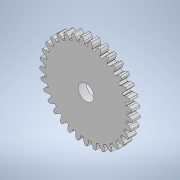
# Autodesk Inventor part: m1歯数33ギア3td6
Saved by Autodesk Inventor 2020.2 (Build 242310000, 310)
## iProperties
Created: 2020-02-29
Part Number: m1歯数33ギア3td6
Material: 一般
Document SubType Name: Modeling
Designer: aoyam
Density: 1 g/cm^3
Appearance: 既定
Author: aoyam
Autodesk Inventor part; units mm, degrees
ref_plane "YZ Plane" through (0, 0, 0) normal (1, 0, 0) x (0, 1, 0)
ref_plane "XZ Plane" through (0, 0, 0) normal (0, 1, 0) x (-1, 0, 0)
ref_plane "XY Plane" through (0, 0, 0) normal (0, 0, 1) x (1, 0, 0)
sketch "スケッチ1" plane through (0, 0, 0) normal (0, 0, 1) x (1, 0, 0)
  arc A0 (1.8965, 18.4525) -> (1.8679, 18.2509) centre (3.2757, 18.1542) ccw
  arc A1 (2.0839, 19.0802) -> (1.8965, 18.4525) centre (5.6844, 17.6636) ccw
  arc A2 (2.6531, 20.2065) -> (2.0839, 19.0802) centre (8.2766, 16.6576) ccw
  arc A3 (0.8542, 18.2509) -> (0.8257, 18.4525) centre (-0.5535, 18.1542) ccw
  arc A4 (0.8257, 18.4525) -> (0.6383, 19.0802) centre (-2.9622, 17.6636) ccw
  arc A5 (0.6383, 19.0802) -> (0.0691, 20.2065) centre (-5.5545, 16.6576) ccw
  arc A6 (1.8596, 17.9961) -> (0.8626, 17.9961) centre (1.3611, 2.7543) ccw
  arc A7 (0.0691, 20.2065) -> (-0.6732, 20.1356) centre (1.3611, 2.7543) ccw
  line L0 (1.8596, 17.9961) -> (1.8679, 18.2509)
  line L1 (0.8626, 17.9961) -> (0.8542, 18.2509)
  arc A8 (-1.0841, 18.2701) -> (-1.074, 18.0668) centre (0.3266, 18.2383) ccw
  arc A9 (-1.034, 17.815) -> (-2.013, 17.6263) centre (1.3611, 2.7543) ccw
  line L2 (-1.034, 17.815) -> (-1.074, 18.0668)
  line L3 (-2.013, 17.6263) -> (-2.0694, 17.8749)
  arc A10 (-2.0694, 17.8749) -> (-2.1356, 18.0675) centre (-3.4334, 17.5136) ccw
  arc A11 (-1.0189, 18.922) -> (-1.0841, 18.2701) centre (2.7846, 18.2124) ccw
  arc A12 (-2.1356, 18.0675) -> (-2.4384, 18.6484) centre (-5.7057, 16.576) ccw
  arc A13 (-0.6732, 20.1356) -> (-1.0189, 18.922) centre (5.5204, 17.7151) ccw
  arc A14 (-2.4384, 18.6484) -> (-3.2104, 19.6466) centre (-8.0607, 15.0976) ccw
  arc A15 (-3.2104, 19.6466) -> (-3.9258, 19.4365) centre (1.3611, 2.7543) ccw
  arc A16 (-3.9763, 17.527) -> (-3.9279, 17.3292) centre (-2.5851, 17.7627) ccw
  arc A17 (-3.8409, 17.0896) -> (-4.7666, 16.719) centre (1.3611, 2.7543) ccw
  line L4 (-3.8409, 17.0896) -> (-3.9279, 17.3292)
  line L5 (-4.7666, 16.719) -> (-4.869, 16.9525)
  arc A18 (-4.869, 16.9525) -> (-4.9704, 17.129) centre (-6.14, 16.3395) ccw
  arc A19 (-4.0356, 18.1794) -> (-3.9763, 17.527) centre (-0.1666, 18.2024) ccw
  arc A20 (-4.9704, 17.129) -> (-5.3777, 17.6421) centre (-8.1938, 14.9888) ccw
  arc A21 (-3.9258, 19.4365) -> (-4.0356, 18.1794) centre (2.6139, 18.2319) ccw
  arc A22 (-5.3777, 17.6421) -> (-6.3247, 18.4762) centre (-10.2265, 13.0914) ccw
  arc A23 (-6.3247, 18.4762) -> (-6.9874, 18.1345) centre (1.3611, 2.7543) ccw
  arc A24 (-6.6756, 16.2499) -> (-6.5907, 16.0649) centre (-5.3541, 16.7446) ccw
  arc A25 (-6.4599, 15.846) -> (-7.2987, 15.307) centre (1.3611, 2.7543) ccw
  line L6 (-6.4599, 15.846) -> (-6.5907, 16.0649)
  line L7 (-7.2987, 15.307) -> (-7.4434, 15.5168)
  arc A26 (-7.4434, 15.5168) -> (-7.5765, 15.671) centre (-8.5754, 14.6744) ccw
  arc A27 (-6.8573, 16.8793) -> (-6.6756, 16.2499) centre (-3.0625, 17.6342) ccw
  arc A28 (-7.5765, 15.671) -> (-8.0734, 16.0977) centre (-10.3365, 12.9595) ccw
  arc A29 (-6.9874, 18.1345) -> (-6.8573, 16.8793) centre (-0.3379, 18.1893) ccw
  arc A30 (-8.0734, 16.0977) -> (-9.1612, 16.7375) centre (-11.9734, 10.7117) ccw
  arc A31 (-9.1612, 16.7375) -> (-9.7473, 16.2766) centre (1.3611, 2.7543) ccw
  arc A32 (-9.0844, 14.4851) -> (-8.966, 14.3195) centre (-7.8805, 15.221) ccw
  arc A33 (-8.7962, 14.1293) -> (-9.5178, 13.4413) centre (1.3611, 2.7543) ccw
  line L8 (-8.7962, 14.1293) -> (-8.966, 14.3195)
  line L9 (-9.5178, 13.4413) -> (-9.6997, 13.6199)
  arc A34 (-9.6997, 13.6199) -> (-9.8594, 13.7461) centre (-10.6518, 12.5785) ccw
  arc A35 (-9.382, 15.0687) -> (-9.0844, 14.4851) centre (-5.7986, 16.5281) ccw
  arc A36 (-9.8594, 13.7461) -> (-10.4282, 14.0711) centre (-12.0565, 10.5613) ccw
  arc A37 (-9.7473, 16.2766) -> (-9.382, 15.0687) centre (-3.2283, 17.5889) ccw
  arc A38 (-10.4282, 14.0711) -> (-11.6174, 14.4935) centre (-13.2384, 8.0443) ccw
  arc A39 (-11.6174, 14.4935) -> (-12.1057, 13.93) centre (1.3611, 2.7543) ccw
  arc A40 (-11.1158, 12.2963) -> (-10.9681, 12.1561) centre (-10.0728, 13.2467) ccw
  arc A41 (-10.7654, 12.0015) -> (-11.3437, 11.1893) centre (1.3611, 2.7543) ccw
  line L10 (-10.7654, 12.0015) -> (-10.9681, 12.1561)
  line L11 (-11.3437, 11.1893) -> (-11.5561, 11.3303)
  arc A42 (-11.5561, 11.3303) -> (-11.7369, 11.424) centre (-12.2939, 10.1275) ccw
  arc A43 (-11.5184, 12.813) -> (-11.1158, 12.2963) centre (-8.276, 14.9242) ccw
  arc A44 (-11.7369, 11.424) -> (-12.3569, 11.6355) centre (-13.2915, 7.8809) ccw
  arc A45 (-12.1057, 13.93) -> (-11.5184, 12.813) centre (-5.9528, 16.4522) ccw
  arc A46 (-12.3569, 11.6355) -> (-13.6045, 11.8251) centre (-13.9757, 5.1858) ccw
  arc A47 (-13.6045, 11.8251) -> (-13.9773, 11.1794) centre (1.3611, 2.7543) ccw
  arc A48 (-12.6961, 9.7626) -> (-12.5246, 9.6528) centre (-11.8519, 10.8932) ccw
  arc A49 (-12.2963, 9.5394) -> (-12.7105, 8.6325) centre (1.3611, 2.7543) ccw
  line L12 (-12.2963, 9.5394) -> (-12.5246, 9.6528)
  line L13 (-12.7105, 8.6325) -> (-12.9457, 8.7308)
  arc A50 (-12.9457, 8.7308) -> (-13.141, 8.7885) centre (-13.4426, 7.4101) ccw
  arc A51 (-13.1893, 10.1938) -> (-12.6961, 9.7626) centre (-10.405, 12.8805) ccw
  arc A52 (-13.141, 8.7885) -> (-13.7898, 8.8788) centre (-13.9969, 5.0152) ccw
  arc A53 (-13.9773, 11.1794) -> (-13.1893, 10.1938) centre (-8.413, 14.8205) ccw
  arc A54 (-13.7898, 8.8788) -> (-15.0508, 8.829) centre (-14.1587, 2.2393) ccw
  arc A55 (-15.0508, 8.829) -> (-15.2946, 8.1243) centre (1.3611, 2.7543) ccw
  arc A56 (-13.7684, 6.9756) -> (-13.5792, 6.9003) centre (-13.1534, 8.2456) ccw
  arc A57 (-13.3336, 6.8321) -> (-13.5687, 5.8632) centre (1.3611, 2.7543) ccw
  line L14 (-13.3336, 6.8321) -> (-13.5792, 6.9003)
  line L15 (-13.5687, 5.8632) -> (-13.8182, 5.9152)
  arc A58 (-13.8182, 5.9152) -> (-14.0209, 5.9349) centre (-14.0562, 4.5243) ccw
  arc A59 (-14.3343, 7.3057) -> (-13.7684, 6.9756) centre (-12.1088, 10.4707) ccw
  arc A60 (-14.0209, 5.9349) -> (-14.6751, 5.9008) centre (-14.1473, 2.0678) ccw
  arc A61 (-15.2946, 8.1243) -> (-14.3343, 7.3057) centre (-10.52, 12.7527) ccw
  arc A62 (-14.6751, 5.9008) -> (-15.9038, 5.6132) centre (-13.7808, -0.6885) ccw
  arc A63 (-15.9038, 5.6132) -> (-16.0099, 4.8752) centre (1.3611, 2.7543) ccw
  arc A64 (-14.2939, 4.036) -> (-14.0939, 3.9979) centre (-13.9303, 5.3994) ccw
  arc A65 (-13.8398, 3.9775) -> (-13.8872, 2.9815) centre (1.3611, 2.7543) ccw
  line L16 (-13.8398, 3.9775) -> (-14.0939, 3.9979)
  line L17 (-13.8872, 2.9815) -> (-14.1421, 2.9853)
  arc A66 (-14.1421, 2.9853) -> (-14.3449, 2.9664) centre (-14.1125, 1.5746) ccw
  arc A67 (-14.912, 4.2531) -> (-14.2939, 4.036) centre (-13.3257, 7.7821) ccw
  arc A68 (-14.3449, 2.9664) -> (-14.9808, 2.8091) centre (-13.7371, -0.8547) ccw
  arc A69 (-16.0099, 4.8752) -> (-14.912, 4.2531) centre (-12.1975, 10.3235) ccw
  arc A70 (-14.9808, 2.8091) -> (-16.1329, 2.2942) centre (-12.8556, -3.4919) ccw
  arc A71 (-16.1329, 2.2942) -> (-16.0974, 1.5494) centre (1.3611, 2.7543) ccw
  arc A72 (-14.2536, 1.0501) -> (-14.05, 1.0506) centre (-14.1546, 2.4577) ccw
  arc A73 (-13.7966, 1.0786) -> (-13.6547, 0.0917) centre (1.3611, 2.7543) ccw
  line L18 (-13.7966, 1.0786) -> (-14.05, 1.0506)
  line L19 (-13.6547, 0.0917) -> (-13.9057, 0.0472)
  arc A74 (-13.9057, 0.0472) -> (-14.1012, -0.0098) centre (-13.6097, -1.3325) ccw
  arc A75 (-14.9016, 1.1463) -> (-14.2536, 1.0501) centre (-14.0118, 4.9117) ccw
  arc A76 (-14.1012, -0.0098) -> (-14.6958, -0.2846) centre (-12.7813, -3.6469) ccw
  arc A77 (-16.0974, 1.5494) -> (-14.9016, 1.1463) centre (-13.3849, 7.6208) ccw
  arc A78 (-14.6958, -0.2846) -> (-15.7297, -1.0083) centre (-11.4166, -6.0696) ccw
  arc A79 (-15.7297, -1.0083) -> (-15.5539, -1.7329) centre (1.3611, 2.7543) ccw
  arc A80 (-13.6489, -1.8742) -> (-13.449, -1.8352) centre (-13.8181, -0.4733) ccw
  arc A81 (-13.2055, -1.7598) -> (-12.8794, -2.702) centre (1.3611, 2.7543) ccw
  line L20 (-13.2055, -1.7598) -> (-13.449, -1.8352)
  line L21 (-12.8794, -2.702) -> (-13.1175, -2.7932)
  arc A82 (-13.1175, -2.7932) -> (-13.2986, -2.8861) centre (-12.5657, -4.0919) ccw
  arc A83 (-14.3034, -1.9024) -> (-13.6489, -1.8742) centre (-14.1423, 1.9634) ccw
  arc A84 (-13.2986, -2.8861) -> (-13.8306, -3.2685) centre (-11.3143, -6.2076) ccw
  arc A85 (-15.5539, -1.7329) -> (-14.3034, -1.9024) centre (-14.0395, 4.7421) ccw
  arc A86 (-13.8306, -3.2685) -> (-14.7087, -4.1747) centre (-9.5157, -8.3283) ccw
  arc A87 (-14.7087, -4.1747) -> (-14.399, -4.853) centre (1.3611, 2.7543) ccw
  arc A88 (-12.5017, -4.6312) -> (-12.3128, -4.5551) centre (-12.933, -3.2876) ccw
  arc A89 (-12.088, -4.4349) -> (-11.5895, -5.2984) centre (1.3611, 2.7543) ccw
  line L22 (-12.088, -4.4349) -> (-12.3128, -4.5551)
  line L23 (-11.5895, -5.2984) -> (-11.806, -5.433)
  arc A90 (-11.806, -5.433) -> (-11.9663, -5.5585) centre (-11.0184, -6.6038) ccw
  arc A91 (-13.139, -4.7828) -> (-12.5017, -4.6312) centre (-13.7125, -0.9563) ccw
  arc A92 (-11.9663, -5.5585) -> (-12.4162, -6.0347) centre (-9.3892, -8.4445) ccw
  arc A93 (-14.399, -4.853) -> (-13.139, -4.7828) centre (-14.1374, 1.7916) ccw
  arc A94 (-12.4162, -6.0347) -> (-13.107, -7.0907) centre (-7.2218, -10.1865) ccw
  arc A95 (-13.107, -7.0907) -> (-12.6745, -7.6981) centre (1.3611, 2.7543) ccw
  arc A96 (-10.8535, -7.1212) -> (-10.6824, -7.0108) centre (-11.5312, -5.8836) ccw
  arc A97 (-10.4844, -6.8503) -> (-9.8315, -7.6038) centre (1.3611, 2.7543) ccw
  line L24 (-10.4844, -6.8503) -> (-10.6824, -7.0108)
  line L25 (-9.8315, -7.6038) -> (-10.0186, -7.7769)
  arc A98 (-10.0186, -7.7769) -> (-10.1522, -7.9305) centre (-9.0236, -8.7775) ccw
  arc A99 (-11.4506, -7.3907) -> (-10.8535, -7.1212) centre (-12.7378, -3.742) ccw
  arc A100 (-10.1522, -7.9305) -> (-10.5039, -8.4832) centre (-7.0755, -10.2766) ccw
  arc A101 (-12.6745, -7.6981) -> (-11.4506, -7.3907) centre (-13.6751, -1.1241) ccw
  arc A102 (-10.5039, -8.4832) -> (-10.9824, -9.6509) centre (-4.6177, -11.5769) ccw
  arc A103 (-10.9824, -9.6509) -> (-10.4428, -10.1655) centre (1.3611, 2.7543) ccw
  arc A104 (-8.7638, -9.2544) -> (-8.6167, -9.1136) centre (-9.6635, -8.1674) ccw
  arc A105 (-8.4527, -8.9185) -> (-7.669, -9.5348) centre (1.3611, 2.7543) ccw
  line L26 (-8.4527, -8.9185) -> (-8.6167, -9.1136)
  line L27 (-7.669, -9.5348) -> (-7.8199, -9.7402)
  arc A106 (-7.8199, -9.7402) -> (-7.9221, -9.9164) centre (-6.6536, -10.5344) ccw
  arc A107 (-9.2991, -9.632) -> (-8.7638, -9.2544) centre (-11.2536, -6.2928) ccw
  arc A108 (-7.9221, -9.9164) -> (-8.1628, -10.5256) centre (-4.4569, -11.6378) ccw
  arc A109 (-10.4428, -10.1655) -> (-9.2991, -9.632) centre (-12.6694, -3.8996) ccw
  arc A110 (-8.1628, -10.5256) -> (-8.4116, -11.7628) centre (-1.7974, -12.4494) ccw
  arc A111 (-8.4116, -11.7628) -> (-7.7844, -12.1659) centre (1.3611, 2.7543) ccw
  arc A112 (-6.3082, -10.9535) -> (-6.1904, -10.7874) centre (-7.3974, -10.0565) ccw
  arc A113 (-6.0662, -10.5648) -> (-5.18, -11.0217) centre (1.3611, 2.7543) ccw
  line L28 (-6.0662, -10.5648) -> (-6.1904, -10.7874)
  line L29 (-5.18, -11.0217) -> (-5.2894, -11.252)
  arc A114 (-5.2894, -11.252) -> (-5.3564, -11.4442) centre (-3.9938, -11.8111) ccw
  arc A115 (-6.7623, -11.4256) -> (-6.3082, -10.9535) centre (-9.3135, -8.5167) ccw
  arc A116 (-5.3564, -11.4442) -> (-5.4775, -12.088) centre (-1.6281, -12.4788) ccw
  arc A117 (-7.7844, -12.1659) -> (-6.7623, -11.4256) centre (-11.1566, -6.4346) ccw
  arc A118 (-5.4775, -12.088) -> (-5.4877, -13.3499) centre (1.137, -12.7724) ccw
  arc A119 (-5.4877, -13.3499) -> (-4.7954, -13.627) centre (1.3611, 2.7543) ccw
  arc A120 (-3.5754, -12.1572) -> (-3.4912, -11.9719) centre (-4.8146, -11.4825) ccw
  arc A121 (-3.4114, -11.7297) -> (-2.4547, -12.0106) centre (1.3611, 2.7543) ccw
  line L30 (-3.4114, -11.7297) -> (-3.4912, -11.9719)
  line L31 (-2.4547, -12.0106) -> (-2.5185, -12.2575)
  arc A122 (-2.5185, -12.2575) -> (-2.5479, -12.4589) centre (-1.1406, -12.5613) ccw
  arc A123 (-3.932, -12.7067) -> (-3.5754, -12.1572) centre (-6.9876, -10.3331) ccw
  arc A124 (-2.5479, -12.4589) -> (-2.545, -13.114) centre (1.3088, -12.7692) ccw
  arc A125 (-4.7954, -13.627) -> (-3.932, -12.7067) centre (-9.1914, -8.6376) ccw
  arc A126 (-2.545, -13.114) -> (-2.3161, -14.355) centre (4.0795, -12.5342) ccw
  arc A127 (-2.3161, -14.355) -> (-1.584, -14.4961) centre (1.3611, 2.7543) ccw
  arc A128 (-0.6641, -12.822) -> (-0.6165, -12.624) centre (-2.0087, -12.394) ccw
  arc A129 (-0.584, -12.3712) -> (0.4085, -12.466) centre (1.3611, 2.7543) ccw
  line L32 (-0.584, -12.3712) -> (-0.6165, -12.624)
  line L33 (0.4085, -12.466) -> (0.3926, -12.7204)
  arc A130 (0.3926, -12.7204) -> (0.4019, -12.9238) centre (1.8031, -12.758) ccw
  arc A131 (-0.9103, -13.429) -> (-0.6641, -12.822) centre (-4.3599, -11.6766) ccw
  arc A132 (0.4019, -12.9238) -> (0.5287, -13.5665) centre (4.2476, -12.4985) ccw
  arc A133 (-1.584, -14.4961) -> (-0.9103, -13.429) centre (-6.8448, -10.4288) ccw
  arc A134 (0.5287, -13.5665) -> (0.9883, -14.7418) centre (6.9237, -11.7435) ccw
  arc A135 (0.9883, -14.7418) -> (1.7339, -14.7418) centre (1.3611, 2.7543) ccw
  arc A136 (2.3203, -12.9238) -> (2.3296, -12.7204) centre (0.919, -12.758) ccw
  arc A137 (2.3136, -12.466) -> (3.3062, -12.3712) centre (1.3611, 2.7543) ccw
  line L34 (2.3136, -12.466) -> (2.3296, -12.7204)
  line L35 (3.3062, -12.3712) -> (3.3387, -12.624)
  arc A138 (3.3387, -12.624) -> (3.3863, -12.822) centre (4.7309, -12.394) ccw
  arc A139 (2.1934, -13.5665) -> (2.3203, -12.9238) centre (-1.5254, -12.4985) ccw
  arc A140 (3.3863, -12.822) -> (3.6325, -13.429) centre (7.082, -11.6766) ccw
  arc A141 (1.7339, -14.7418) -> (2.1934, -13.5665) centre (-4.2016, -11.7435) ccw
  arc A142 (3.6325, -13.429) -> (4.3061, -14.4961) centre (9.5669, -10.4288) ccw
  arc A143 (4.3061, -14.4961) -> (5.0383, -14.355) centre (1.3611, 2.7543) ccw
  arc A144 (5.27, -12.4589) -> (5.2407, -12.2575) centre (3.8627, -12.5613) ccw
  arc A145 (5.1769, -12.0106) -> (6.1335, -11.7297) centre (1.3611, 2.7543) ccw
  line L36 (5.1769, -12.0106) -> (5.2407, -12.2575)
  line L37 (6.1335, -11.7297) -> (6.2133, -11.9719)
  arc A146 (6.2133, -11.9719) -> (6.2975, -12.1572) centre (7.5368, -11.4825) ccw
  arc A147 (5.2671, -13.114) -> (5.27, -12.4589) centre (1.4133, -12.7692) ccw
  arc A148 (6.2975, -12.1572) -> (6.6541, -12.7067) centre (9.7097, -10.3331) ccw
  arc A149 (5.0383, -14.355) -> (5.2671, -13.114) centre (-1.3573, -12.5342) ccw
  arc A150 (6.6541, -12.7067) -> (7.5176, -13.627) centre (11.9135, -8.6376) ccw
  arc A151 (7.5176, -13.627) -> (8.2098, -13.3499) centre (1.3611, 2.7543) ccw
  arc A152 (8.0785, -11.4442) -> (8.0115, -11.252) centre (6.716, -11.8111) ccw
  arc A153 (7.9022, -11.0217) -> (8.7884, -10.5648) centre (1.3611, 2.7543) ccw
  line L38 (7.9022, -11.0217) -> (8.0115, -11.252)
  line L39 (8.7884, -10.5648) -> (8.9126, -10.7874)
  arc A154 (8.9126, -10.7874) -> (9.0303, -10.9535) centre (10.1195, -10.0565) ccw
  arc A155 (8.1996, -12.088) -> (8.0785, -11.4442) centre (4.3502, -12.4788) ccw
  arc A156 (9.0303, -10.9535) -> (9.4845, -11.4256) centre (12.0356, -8.5167) ccw
  arc A157 (8.2098, -13.3499) -> (8.1996, -12.088) centre (1.5852, -12.7724) ccw
  arc A158 (9.4845, -11.4256) -> (10.5065, -12.1659) centre (13.8787, -6.4346) ccw
  arc A159 (10.5065, -12.1659) -> (11.1338, -11.7628) centre (1.3611, 2.7543) ccw
  arc A160 (10.6442, -9.9164) -> (10.542, -9.7402) centre (9.3757, -10.5344) ccw
  arc A161 (10.3911, -9.5348) -> (11.1748, -8.9185) centre (1.3611, 2.7543) ccw
  line L40 (10.3911, -9.5348) -> (10.542, -9.7402)
  line L41 (11.1748, -8.9185) -> (11.3389, -9.1136)
  arc A162 (11.3389, -9.1136) -> (11.4859, -9.2544) centre (12.3857, -8.1674) ccw
  arc A163 (10.8849, -10.5256) -> (10.6442, -9.9164) centre (7.1791, -11.6378) ccw
  arc A164 (11.4859, -9.2544) -> (12.0213, -9.632) centre (13.9758, -6.2928) ccw
  arc A165 (11.1338, -11.7628) -> (10.8849, -10.5256) centre (4.5196, -12.4494) ccw
  arc A166 (12.0213, -9.632) -> (13.1649, -10.1655) centre (15.3915, -3.8996) ccw
  arc A167 (13.1649, -10.1655) -> (13.7045, -9.6509) centre (1.3611, 2.7543) ccw
  arc A168 (12.8744, -7.9305) -> (12.7407, -7.7769) centre (11.7458, -8.7775) ccw
  arc A169 (12.5536, -7.6038) -> (13.2066, -6.8503) centre (1.3611, 2.7543) ccw
  line L42 (12.5536, -7.6038) -> (12.7407, -7.7769)
  line L43 (13.2066, -6.8503) -> (13.4046, -7.0108)
  arc A170 (13.4046, -7.0108) -> (13.5756, -7.1212) centre (14.2534, -5.8836) ccw
  arc A171 (13.2261, -8.4832) -> (12.8744, -7.9305) centre (9.7977, -10.2766) ccw
  arc A172 (13.5756, -7.1212) -> (14.1727, -7.3907) centre (15.46, -3.742) ccw
  arc A173 (13.7045, -9.6509) -> (13.2261, -8.4832) centre (7.3398, -11.5769) ccw
  arc A174 (14.1727, -7.3907) -> (15.3967, -7.6981) centre (16.3972, -1.1241) ccw
  arc A175 (15.3967, -7.6981) -> (15.8292, -7.0907) centre (1.3611, 2.7543) ccw
  arc A176 (14.6884, -5.5585) -> (14.5281, -5.433) centre (13.7405, -6.6038) ccw
  arc A177 (14.3116, -5.2984) -> (14.8102, -4.4349) centre (1.3611, 2.7543) ccw
  line L44 (14.3116, -5.2984) -> (14.5281, -5.433)
  line L45 (14.8102, -4.4349) -> (15.035, -4.5551)
  arc A178 (15.035, -4.5551) -> (15.2239, -4.6312) centre (15.6551, -3.2876) ccw
  arc A179 (15.1384, -6.0347) -> (14.6884, -5.5585) centre (12.1113, -8.4445) ccw
  arc A180 (15.2239, -4.6312) -> (15.8612, -4.7828) centre (16.4346, -0.9563) ccw
  arc A181 (15.8292, -7.0907) -> (15.1384, -6.0347) centre (9.9439, -10.1865) ccw
  arc A182 (15.8612, -4.7828) -> (17.1211, -4.853) centre (16.8595, 1.7916) ccw
  arc A183 (17.1211, -4.853) -> (17.4309, -4.1747) centre (1.3611, 2.7543) ccw
  arc A184 (16.0208, -2.8861) -> (15.8396, -2.7932) centre (15.2878, -4.0919) ccw
  arc A185 (15.6016, -2.702) -> (15.9277, -1.7598) centre (1.3611, 2.7543) ccw
  line L46 (15.6016, -2.702) -> (15.8396, -2.7932)
  line L47 (15.9277, -1.7598) -> (16.1712, -1.8352)
  arc A186 (16.1712, -1.8352) -> (16.371, -1.8742) centre (16.5403, -0.4733) ccw
  arc A187 (16.5527, -3.2685) -> (16.0208, -2.8861) centre (14.0364, -6.2076) ccw
  arc A188 (16.371, -1.8742) -> (17.0255, -1.9024) centre (16.8644, 1.9634) ccw
  arc A189 (17.4309, -4.1747) -> (16.5527, -3.2685) centre (12.2379, -8.3283) ccw
  arc A190 (17.0255, -1.9024) -> (18.276, -1.7329) centre (16.7616, 4.7421) ccw
  arc A191 (18.276, -1.7329) -> (18.4518, -1.0083) centre (1.3611, 2.7543) ccw
  arc A192 (16.8233, -0.0098) -> (16.6278, 0.0472) centre (16.3318, -1.3325) ccw
  arc A193 (16.3768, 0.0917) -> (16.5187, 1.0786) centre (1.3611, 2.7543) ccw
  line L48 (16.3768, 0.0917) -> (16.6278, 0.0472)
  line L49 (16.5187, 1.0786) -> (16.7721, 1.0506)
  arc A194 (16.7721, 1.0506) -> (16.9757, 1.0501) centre (16.8768, 2.4577) ccw
  arc A195 (17.418, -0.2846) -> (16.8233, -0.0098) centre (15.5034, -3.6469) ccw
  arc A196 (16.9757, 1.0501) -> (17.6237, 1.1463) centre (16.734, 4.9117) ccw
  arc A197 (18.4518, -1.0083) -> (17.418, -0.2846) centre (14.1387, -6.0696) ccw
  arc A198 (17.6237, 1.1463) -> (18.8195, 1.5494) centre (16.1071, 7.6208) ccw
  arc A199 (18.8195, 1.5494) -> (18.855, 2.2942) centre (1.3611, 2.7543) ccw
  arc A200 (17.067, 2.9664) -> (16.8643, 2.9853) centre (16.8347, 1.5746) ccw
  arc A201 (16.6094, 2.9815) -> (16.5619, 3.9775) centre (1.3611, 2.7543) ccw
  line L50 (16.6094, 2.9815) -> (16.8643, 2.9853)
  line L51 (16.5619, 3.9775) -> (16.816, 3.9979)
  arc A202 (16.816, 3.9979) -> (17.016, 4.036) centre (16.6525, 5.3994) ccw
  arc A203 (17.7029, 2.8091) -> (17.067, 2.9664) centre (16.4593, -0.8547) ccw
  arc A204 (17.016, 4.036) -> (17.6341, 4.2531) centre (16.0478, 7.7821) ccw
  arc A205 (18.855, 2.2942) -> (17.7029, 2.8091) centre (15.5777, -3.4919) ccw
  arc A206 (17.6341, 4.2531) -> (18.7321, 4.8752) centre (14.9196, 10.3235) ccw
  arc A207 (18.7321, 4.8752) -> (18.626, 5.6132) centre (1.3611, 2.7543) ccw
  arc A208 (16.743, 5.9349) -> (16.5404, 5.9152) centre (16.7783, 4.5243) ccw
  arc A209 (16.2908, 5.8632) -> (16.0557, 6.8321) centre (1.3611, 2.7543) ccw
  line L52 (16.2908, 5.8632) -> (16.5404, 5.9152)
  line L53 (16.0557, 6.8321) -> (16.3014, 6.9003)
  arc A210 (16.3014, 6.9003) -> (16.4906, 6.9756) centre (15.8756, 8.2456) ccw
  arc A211 (17.3972, 5.9008) -> (16.743, 5.9349) centre (16.8694, 2.0678) ccw
  arc A212 (16.4906, 6.9756) -> (17.0564, 7.3057) centre (14.8309, 10.4707) ccw
  arc A213 (18.626, 5.6132) -> (17.3972, 5.9008) centre (16.5029, -0.6885) ccw
  arc A214 (17.0564, 7.3057) -> (18.0168, 8.1243) centre (13.2421, 12.7527) ccw
  arc A215 (18.0168, 8.1243) -> (17.7729, 8.829) centre (1.3611, 2.7543) ccw
  arc A216 (15.8631, 8.7885) -> (15.6679, 8.7308) centre (16.1647, 7.4101) ccw
  arc A217 (15.4326, 8.6325) -> (15.0185, 9.5394) centre (1.3611, 2.7543) ccw
  line L54 (15.4326, 8.6325) -> (15.6679, 8.7308)
  line L55 (15.0185, 9.5394) -> (15.2468, 9.6528)
  arc A218 (15.2468, 9.6528) -> (15.4183, 9.7626) centre (14.574, 10.8932) ccw
  arc A219 (16.5119, 8.8788) -> (15.8631, 8.7885) centre (16.7191, 5.0152) ccw
  arc A220 (15.4183, 9.7626) -> (15.9114, 10.1938) centre (13.1271, 12.8805) ccw
  arc A221 (17.7729, 8.829) -> (16.5119, 8.8788) centre (16.8808, 2.2393) ccw
  arc A222 (15.9114, 10.1938) -> (16.6995, 11.1794) centre (11.1352, 14.8205) ccw
  arc A223 (16.6995, 11.1794) -> (16.3267, 11.8251) centre (1.3611, 2.7543) ccw
  arc A224 (14.459, 11.424) -> (14.2783, 11.3303) centre (15.0161, 10.1275) ccw
  arc A225 (14.0659, 11.1893) -> (13.4875, 12.0015) centre (1.3611, 2.7543) ccw
  line L56 (14.0659, 11.1893) -> (14.2783, 11.3303)
  line L57 (13.4875, 12.0015) -> (13.6903, 12.1561)
  arc A226 (13.6903, 12.1561) -> (13.8379, 12.2963) centre (12.7949, 13.2467) ccw
  arc A227 (15.0791, 11.6355) -> (14.459, 11.424) centre (16.0136, 7.8809) ccw
  arc A228 (13.8379, 12.2963) -> (14.2405, 12.813) centre (10.9981, 14.9242) ccw
  arc A229 (16.3267, 11.8251) -> (15.0791, 11.6355) centre (16.6978, 5.1858) ccw
  arc A230 (14.2405, 12.813) -> (14.8278, 13.93) centre (8.675, 16.4522) ccw
  arc A231 (14.8278, 13.93) -> (14.3395, 14.4935) centre (1.3611, 2.7543) ccw
  arc A232 (12.5816, 13.7461) -> (12.4218, 13.6199) centre (13.3739, 12.5785) ccw
  arc A233 (12.2399, 13.4413) -> (11.5184, 14.1293) centre (1.3611, 2.7543) ccw
  line L58 (12.2399, 13.4413) -> (12.4218, 13.6199)
  line L59 (11.5184, 14.1293) -> (11.6882, 14.3195)
  arc A234 (11.6882, 14.3195) -> (11.8066, 14.4851) centre (10.6026, 15.221) ccw
  arc A235 (13.1504, 14.0711) -> (12.5816, 13.7461) centre (14.7786, 10.5613) ccw
  arc A236 (11.8066, 14.4851) -> (12.1042, 15.0687) centre (8.5208, 16.5281) ccw
  arc A237 (14.3395, 14.4935) -> (13.1504, 14.0711) centre (15.9605, 8.0443) ccw
  arc A238 (12.1042, 15.0687) -> (12.4695, 16.2766) centre (5.9505, 17.5889) ccw
  arc A239 (12.4695, 16.2766) -> (11.8834, 16.7375) centre (1.3611, 2.7543) ccw
  arc A240 (10.2986, 15.671) -> (10.1656, 15.5168) centre (11.2976, 14.6744) ccw
  arc A241 (10.0208, 15.307) -> (9.1821, 15.846) centre (1.3611, 2.7543) ccw
  line L60 (10.0208, 15.307) -> (10.1656, 15.5168)
  line L61 (9.1821, 15.846) -> (9.3128, 16.0649)
  arc A242 (9.3128, 16.0649) -> (9.3978, 16.2499) centre (8.0763, 16.7446) ccw
  arc A243 (10.7956, 16.0977) -> (10.2986, 15.671) centre (13.0587, 12.9595) ccw
  arc A244 (9.3978, 16.2499) -> (9.5795, 16.8793) centre (5.7847, 17.6342) ccw
  arc A245 (11.8834, 16.7375) -> (10.7956, 16.0977) centre (14.6955, 10.7117) ccw
  arc A246 (9.5795, 16.8793) -> (9.7096, 18.1345) centre (3.0601, 18.1893) ccw
  arc A247 (9.7096, 18.1345) -> (9.0468, 18.4762) centre (1.3611, 2.7543) ccw
  arc A248 (7.6926, 17.129) -> (7.5911, 16.9525) centre (8.8621, 16.3395) ccw
  arc A249 (7.4887, 16.719) -> (6.5631, 17.0896) centre (1.3611, 2.7543) ccw
  line L62 (7.4887, 16.719) -> (7.5911, 16.9525)
  line L63 (6.5631, 17.0896) -> (6.65, 17.3292)
  arc A250 (6.65, 17.3292) -> (6.6985, 17.527) centre (5.3072, 17.7627) ccw
  arc A251 (8.0998, 17.6421) -> (7.6926, 17.129) centre (10.9159, 14.9888) ccw
  arc A252 (6.6985, 17.527) -> (6.7578, 18.1794) centre (2.8887, 18.2024) ccw
  arc A253 (9.0468, 18.4762) -> (8.0998, 17.6421) centre (12.9486, 13.0914) ccw
  arc A254 (6.7578, 18.1794) -> (6.648, 19.4365) centre (0.1082, 18.2319) ccw
  arc A255 (6.648, 19.4365) -> (5.9326, 19.6466) centre (1.3611, 2.7543) ccw
  arc A256 (4.8577, 18.0675) -> (4.7915, 17.8749) centre (6.1555, 17.5136) ccw
  arc A257 (4.7351, 17.6263) -> (3.7561, 17.815) centre (1.3611, 2.7543) ccw
  line L64 (4.7351, 17.6263) -> (4.7915, 17.8749)
  line L65 (3.7561, 17.815) -> (3.7961, 18.0668)
  arc A258 (3.7961, 18.0668) -> (3.8062, 18.2701) centre (2.3955, 18.2383) ccw
  arc A259 (5.1605, 18.6484) -> (4.8577, 18.0675) centre (8.4279, 16.576) ccw
  arc A260 (3.8062, 18.2701) -> (3.741, 18.922) centre (-0.0625, 18.2124) ccw
  arc A261 (5.9326, 19.6466) -> (5.1605, 18.6484) centre (10.7829, 15.0976) ccw
  arc A262 (3.741, 18.922) -> (3.3953, 20.1356) centre (-2.7983, 17.7151) ccw
  arc A263 (3.3953, 20.1356) -> (2.6531, 20.2065) centre (1.3611, 2.7543) ccw
  circle A264 centre (1.3611, 2.7543) radius 3
  point P0 (0, 0)
  point P1 (3.7961, 18.0668)
  point P2 (3.8062, 18.2701)
  point P3 (3.741, 18.922)
  point P4 (3.3953, 20.1356)
  point P5 (2.6531, 20.2065)
  point P6 (2.0839, 19.0802)
  point P7 (1.8965, 18.4525)
  point P8 (1.8679, 18.2509)
  point P9 (1.8596, 17.9961)
  point P10 (0.8626, 17.9961)
  point P11 (0.8542, 18.2509)
  point P12 (0.8257, 18.4525)
  point P13 (0.6383, 19.0802)
  point P14 (0.0691, 20.2065)
  point P15 (-0.6732, 20.1356)
  point P16 (-1.0189, 18.922)
  point P17 (-1.0841, 18.2701)
  point P18 (-1.034, 17.815)
  point P19 (-2.013, 17.6263)
  point P20 (-2.1356, 18.0675)
  point P21 (-2.4384, 18.6484)
  point P22 (-3.2104, 19.6466)
  point P23 (-3.9258, 19.4365)
  point P24 (-4.0356, 18.1794)
  point P25 (-3.9763, 17.527)
  point P26 (-3.9279, 17.3292)
  point P27 (-3.8409, 17.0896)
  point P28 (-4.9704, 17.129)
  point P29 (-5.3777, 17.6421)
  point P30 (-6.3247, 18.4762)
  point P31 (-6.9874, 18.1345)
  point P32 (-6.8573, 16.8793)
  point P33 (-6.6756, 16.2499)
  point P34 (-6.5907, 16.0649)
  point P35 (-6.4599, 15.846)
  point P36 (-7.4434, 15.5168)
  point P37 (-7.5765, 15.671)
  point P38 (-8.0734, 16.0977)
  point P39 (-9.1612, 16.7375)
  point P40 (-9.7473, 16.2766)
  point P41 (-9.382, 15.0687)
  point P42 (-9.0844, 14.4851)
  point P43 (-8.966, 14.3195)
  point P44 (-9.8594, 13.7461)
  point P45 (-10.4282, 14.0711)
  point P46 (-11.6174, 14.4935)
  point P47 (-12.1057, 13.93)
  point P48 (-11.5184, 12.813)
  point P49 (-11.1158, 12.2963)
  point P50 (-10.7654, 12.0015)
  point P51 (-11.3437, 11.1893)
  point P52 (-11.5561, 11.3303)
  point P53 (-11.7369, 11.424)
  point P54 (-12.3569, 11.6355)
  point P55 (-13.6045, 11.8251)
  point P56 (-13.9773, 11.1794)
  point P57 (-13.1893, 10.1938)
  point P58 (-12.6961, 9.7626)
  point P59 (-12.7105, 8.6325)
  point P60 (-13.141, 8.7885)
  point P61 (-13.7898, 8.8788)
  point P62 (-15.0508, 8.829)
  point P63 (-15.2946, 8.1243)
  point P64 (-14.3343, 7.3057)
  point P65 (-13.7684, 6.9756)
  point P66 (-13.3336, 6.8321)
  point P67 (-14.0209, 5.9349)
  point P68 (-14.6751, 5.9008)
  point P69 (-15.9038, 5.6132)
  point P70 (-16.0099, 4.8752)
  point P71 (-14.912, 4.2531)
  point P72 (-14.2939, 4.036)
  point P73 (-14.0939, 3.9979)
  point P74 (-13.8398, 3.9775)
  point P75 (-13.8872, 2.9815)
  point P76 (-14.1421, 2.9853)
  point P77 (-14.3449, 2.9664)
  point P78 (-14.9808, 2.8091)
  point P79 (-16.1329, 2.2942)
  point P80 (-16.0974, 1.5494)
  point P81 (-14.9016, 1.1463)
  point P82 (-14.2536, 1.0501)
  point P83 (-13.7966, 1.0786)
  point P84 (-13.6547, 0.0917)
  point P85 (-13.9057, 0.0472)
  point P86 (-14.1012, -0.0098)
  point P87 (-14.6958, -0.2846)
  point P88 (-15.7297, -1.0083)
  point P89 (-15.5539, -1.7329)
  point P90 (-14.3034, -1.9024)
  point P91 (-13.6489, -1.8742)
  point P92 (-13.449, -1.8352)
  point P93 (-13.2055, -1.7598)
  point P94 (-12.8794, -2.702)
  point P95 (-13.1175, -2.7932)
  point P96 (-13.2986, -2.8861)
  point P97 (-13.8306, -3.2685)
  point P98 (-14.7087, -4.1747)
  point P99 (-14.399, -4.853)
  point P100 (-13.139, -4.7828)
  point P101 (-12.5017, -4.6312)
  point P102 (-12.088, -4.4349)
  point P103 (-11.5895, -5.2984)
  point P104 (-11.806, -5.433)
  point P105 (-11.9663, -5.5585)
  point P106 (-12.4162, -6.0347)
  point P107 (-13.107, -7.0907)
  point P108 (-12.6745, -7.6981)
  point P109 (-11.4506, -7.3907)
  point P110 (-10.8535, -7.1212)
  point P111 (-10.0186, -7.7769)
  point P112 (-10.1522, -7.9305)
  point P113 (-10.5039, -8.4832)
  point P114 (-10.4428, -10.1655)
  point P115 (-9.2991, -9.632)
  point P116 (-8.7638, -9.2544)
  point P117 (-8.6167, -9.1136)
  point P118 (-7.669, -9.5348)
  point P119 (-7.8199, -9.7402)
  point P120 (-7.9221, -9.9164)
  point P121 (-8.1628, -10.5256)
  point P122 (-8.4116, -11.7628)
  point P123 (-7.7844, -12.1659)
  point P124 (-6.7623, -11.4256)
  point P125 (-6.3082, -10.9535)
  point P126 (-5.3564, -11.4442)
  point P127 (-5.4775, -12.088)
  point P128 (-5.4877, -13.3499)
  point P129 (-4.7954, -13.627)
  point P130 (-3.932, -12.7067)
  point P131 (-3.5754, -12.1572)
  point P132 (-3.4912, -11.9719)
  point P133 (-3.4114, -11.7297)
  point P134 (-2.4547, -12.0106)
  point P135 (-2.5479, -12.4589)
  point P136 (-2.545, -13.114)
  point P137 (-2.3161, -14.355)
  point P138 (-1.584, -14.4961)
  point P139 (-0.9103, -13.429)
  point P140 (-0.6641, -12.822)
  point P141 (0.4085, -12.466)
  point P142 (0.4019, -12.9238)
  point P143 (0.5287, -13.5665)
  point P144 (0.9883, -14.7418)
  point P145 (1.7339, -14.7418)
  point P146 (2.1934, -13.5665)
  point P147 (2.3203, -12.9238)
  point P148 (2.3296, -12.7204)
  point P149 (2.3136, -12.466)
  point P150 (3.3062, -12.3712)
  point P151 (3.3387, -12.624)
  point P152 (3.3863, -12.822)
  point P153 (3.6325, -13.429)
  point P154 (4.3061, -14.4961)
  point P155 (5.0383, -14.355)
  point P156 (5.2671, -13.114)
  point P157 (5.27, -12.4589)
  point P158 (5.2407, -12.2575)
  point P159 (5.1769, -12.0106)
  point P160 (6.1335, -11.7297)
  point P161 (6.2133, -11.9719)
  point P162 (6.2975, -12.1572)
  point P163 (6.6541, -12.7067)
  point P164 (7.5176, -13.627)
  point P165 (8.2098, -13.3499)
  point P166 (8.1996, -12.088)
  point P167 (8.0785, -11.4442)
  point P168 (7.9022, -11.0217)
  point P169 (8.7884, -10.5648)
  point P170 (9.0303, -10.9535)
  point P171 (9.4845, -11.4256)
  point P172 (10.5065, -12.1659)
  point P173 (11.1338, -11.7628)
  point P174 (10.8849, -10.5256)
  point P175 (10.6442, -9.9164)
  point P176 (11.1748, -8.9185)
  point P177 (11.3389, -9.1136)
  point P178 (11.4859, -9.2544)
  point P179 (12.0213, -9.632)
  point P180 (13.1649, -10.1655)
  point P181 (13.7045, -9.6509)
  point P182 (13.2261, -8.4832)
  point P183 (12.8744, -7.9305)
  point P184 (12.5536, -7.6038)
  point P185 (13.2066, -6.8503)
  point P186 (13.4046, -7.0108)
  point P187 (13.5756, -7.1212)
  point P188 (14.1727, -7.3907)
  point P189 (15.3967, -7.6981)
  point P190 (15.8292, -7.0907)
  point P191 (15.1384, -6.0347)
  point P192 (14.6884, -5.5585)
  point P193 (15.2239, -4.6312)
  point P194 (15.8612, -4.7828)
  point P195 (17.1211, -4.853)
  point P196 (17.4309, -4.1747)
  point P197 (16.5527, -3.2685)
  point P198 (16.0208, -2.8861)
  point P199 (15.8396, -2.7932)
  dimension "d2" = 360
  dimension "d6" = 6
  constraints: 528 point on circle, 265 centre point, 132 end point, 3 coincident, 1253 other
  measures "d6" diameter of A264
extrude "押し出し1" add sketch "スケッチ1" along normal blind 3
